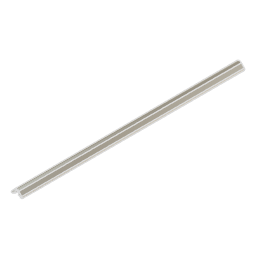
cable-cover-source-fusion (Autodesk Fusion 360 design; units mm, degrees)
Autodesk Fusion 360 part; units mm, degrees
sketch "Sketch1" plane through (0, 0, 0) normal (0, 1, 0) x (1, 0, 0) in component "Main"
  arc A0 (-1.9148, -3.3588) -> (1.9148, -3.3588) centre (0, -1.6) ccw
  line L0 (-1.9148, -3.3588) -> (-5, 0)
  line L1 (1.9148, -3.3588) -> (5, 0)
  line L2 (-5, 0) -> (5, 0)
  line L3 (0, -1.6) -> (0, 0) construction
  circle A1 centre (0, -1.6) radius 1.5 construction
  arc A2 (-1.6, -1.6) -> (1.6, -1.6) centre (0, -1.6) ccw
  line L4 (-1.6, -1.6) -> (-1.6, 0)
  line L5 (1.6, -1.6) -> (1.6, 0)
  point P0 (0, -0.1)
  dimension "d3" = 0.1
  dimension "d4" = 3
  dimension "d5" = 0.1
  dimension "d6" = 1
  dimension "d7" = 85.137
  dimension "d12" = 10
  constraint horizontal L2
  constraint tangent A0 L0
  constraint tangent A0 L1
  constraint midpoint L3.end L2
  constraint coincident L3.end origin
  constraint vertical L3
  constraint coincident L3 P0
  constraint concentric A0 A1
  constraint coincident A0.centre L3.start
  constraint coincident L2 L4.end
  constraint coincident L2 L5.end
  constraint vertical L4
  constraint vertical L5
  constraint tangent A2 L4
  constraint tangent A2 L5
  constraint coincident P0 A1
  measures "d3" distance of L3.end P0
  measures "d4" diameter of A1
  measures "d5" distance of A1 A2
  measures "d6" distance of A0 A2
  measures "d7" angle of L0 L1
  measures "d12" distance of L0.end L1.end
extrude "Extrude1" add sketch "Sketch1" along normal mid plane 200 contours A0 L0 L1 L2 A2 L4 L5 in component "Main"
sketch "Sketch2" plane through (0, 0, 0) normal (0, 0, 1) x (1, 0, 0) in component "Main"
  line L0 (-5, -100) -> (-5, 100)
  line L1 (5, -100) -> (5, 100)
  line L2 (3, -100) -> (-3, -100)
  line L3 (-3, -100) -> (-3, -74.6)
  line L4 (-3, -74.6) -> (3, -74.6)
  line L5 (3, -74.6) -> (3, -100)
  line L6 (-5, -100) -> (3, -74.6) construction
  line L7 (5, -100) -> (-3, -74.6) construction
  line L8 (3, 100) -> (-3, 100)
  line L9 (-3, 100) -> (-3, 74.6)
  line L10 (-3, 74.6) -> (3, 74.6)
  line L11 (3, 74.6) -> (3, 100)
  line L12 (3, -12.7) -> (-3, -12.7)
  line L13 (-3, -12.7) -> (-3, 12.7)
  line L14 (-3, 12.7) -> (3, 12.7)
  line L15 (3, 12.7) -> (3, -12.7)
  line L16 (3, 0) -> (-3, 0) construction
  line L17 (-5, -100) -> (-3, -100)
  line L18 (5, -100) -> (3, -100)
  line L19 (5, 100) -> (3, 100)
  line L20 (-3, 100) -> (-5, 100)
  line L21 (1.6, -100) -> (1.6, 100)
  line L22 (-1.6, -100) -> (-1.6, 100)
  dimension "d17" = 25.4
  dimension "d18" = 2
  dimension "d19" = 25.4
  dimension "d20" = 25.4
  constraint horizontal L2
  constraint vertical L3
  constraint horizontal L4
  constraint vertical L5
  constraint coincident L1.start L2
  constraint coincident L0.start L6.start
  constraint coincident L1.start L7.start
  constraint equal L6 L7
  constraint horizontal L8
  constraint vertical L9
  constraint horizontal L10
  constraint vertical L11
  constraint coincident L1.end L8
  constraint collinear L5 L11
  constraint collinear L3 L9
  constraint horizontal L12
  constraint vertical L13
  constraint horizontal L14
  constraint vertical L15
  constraint midpoint L15 L16.start
  constraint midpoint L13 L16.end
  constraint coincident origin L16
  constraint collinear L5 L15
  constraint collinear L3 L13
  constraint coincident L1.end L19.start
  constraint coincident L0.end L20.end
  measures "d17" distance of L2.start L4.end
  measures "d18" distance of L1 L5
  measures "d19" distance of L8.start L10.end
  measures "d20" distance of L12.start L14.end
extrude "Extrude2" add sketch "Sketch2" against normal blind 0.8 contours L0 L3 L4 L9 L10 L12 L13 L14 L17 L20 L22 | L1 L4 L5 L10 L11 L12 L14 L15 L18 L19 L21 in component "Main"
sketch "Sketch3" plane through (0, 0, 0) normal (0, 1, 0) x (1, 0, 0) in component "Main"
  line L0 (-5, 0) -> (-1.9148, -3.3588)
  line L1 (-5, 0.8) -> (-5, 0)
  arc A0 (-5, 0.8) -> (-4.4588, -0.5892) centre (-2.9464, 0.8) ccw
  line L2 (-5, 0.8) -> (-3, 0.8)
  dimension "d23" = 2.0536
  constraint coincident L1.start A0.start
  constraint coincident A0.centre L2
  constraint coincident L0 A0.end
  constraint tangent L0 A0
  measures "d23" radius of A0
fillet "Fillet1" radius 2.0536 2 edges at (-5, 0, 0) (5, 0, 0) in component "Main"
split "Split1" [suppressed] in component "Main"
extrude "Extrude3" [suppressed] in component "Main"
component "Main" placed x (1, 0, 0) y (0, 1, 0) z (0, 0, 1) at (0, 0, 0)
equation "d4 = CableDiameter"
equation "CableDiameter = 3 mm"
equation "BotWidth = 10 mm"
equation "d12 = BotWidth"
equation "GapWidth = 25.4 mm"
equation "d17 = GapWidth"
equation "d19 = GapWidth"
equation "d20 = GapWidth"
equation "d25 = d23"
